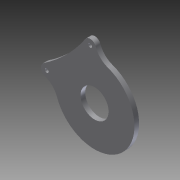
# Autodesk Inventor part: motor plate
Saved by Autodesk Inventor 2012 (Build 160160000, 160)
## iProperties
Created: 2012-02-08
Part Number: motor plate
Material: Default
Document SubType Name: Modeling
Designer: Antonella Wilby
Density: 1 g/cm^3
Author: Antonella Wilby
Autodesk Inventor part; units mm, degrees
ref_plane "YZ Plane" through (0, 0, 0) normal (1, 0, 0) x (0, 1, 0)
ref_plane "XZ Plane" through (0, 0, 0) normal (0, 1, 0) x (-1, 0, 0)
ref_plane "XY Plane" through (0, 0, 0) normal (0, 0, 1) x (1, 0, 0)
sketch "Sketch1" plane through (0, 0, 0) normal (0, 0, 1) x (1, 0, 0)
  line L0 (-237.7169, 0) -> (128.6737, 0) projected
  line L1 (0, -128.6737) -> (0, 237.7169) projected
  line L2 (0, 0) -> (-137.5064, 137.5064) construction
  circle A0 centre (0, 0) radius 19.05
  line L3 (-64.8097, 6.007) -> (-6.007, 64.8097) construction
  line L4 (0, 0) -> (-6.007, 64.8097) construction
  line L5 (0, 0) -> (-64.8097, 6.007) construction
  arc A1 (1.4866, 67.427) -> (-12.5946, 69.2377) centre (-6.007, 64.8097) ccw
  arc A2 (-69.2377, 12.5946) -> (-67.427, -1.4866) centre (-64.8097, 6.007) ccw
  circle A3 centre (-6.007, 64.8097) radius 6.35 construction
  circle A4 centre (-64.8097, 6.007) radius 6.35 construction
  arc A5 (-38.1661, 38.1661) -> (-12.5946, 69.2377) centre (-185.3754, 185.3754) ccw
  arc A6 (1.4866, 67.427) -> (17.9617, 50.8987) centre (26.9305, 76.3138) ccw
  arc A7 (-69.2377, 12.5946) -> (-38.1661, 38.1661) centre (-185.3754, 185.3754) ccw
  arc A8 (-50.8987, -17.9617) -> (-67.427, -1.4866) centre (-76.3138, -26.9305) ccw
  arc A9 (-50.8987, -17.9617) -> (17.9617, 50.8987) centre (0, 0) ccw
  point P0 (-35.4084, 35.4084)
  dimension "d1" = 45
  dimension "d2" = 38.1
  dimension "d3" = 83.1596
  dimension "d5" = 65.0875
  dimension "d6" = 12.7
  dimension "d7" = 1.5875
  dimension "d9" = 53.975
  constraints: 14 point on circle, 10 centre point, 8 coincident, 8 end point, 5 tangent, 2 equal radius, 2 point on line, 1 midpoint, 1 perpendicular, 2 other
  measures "d1" angle of L1 L2
  measures "d2" diameter of A0
  measures "d3" distance of L4.end L5.end
  measures "d5" distance of L4.start L4.end
  measures "d6" diameter of A3
  measures "d7" radial gap between concentric circles of A2 A4
  measures "d9" distance of A5.start point (0, 0)
extrude "Base" add sketch "Sketch1" along normal mid plane 6.35 contours A2 A7 A5 A1 L1 A0 L0 | L0 A0 L1 A9 A8 A2 | L1 A1 A6 A9 L0 A0 | A0 L0 A9 L1
sketch "Sketch2" plane through (0, 0, -3.175) normal (0, 0, -1) x (-1, 0, 0)
  arc A0 (12.5946, 69.2377) -> (-1.4866, 67.427) centre (6.007, 64.8097) ccw projected
  arc A1 (67.427, -1.4866) -> (69.2377, 12.5946) centre (64.8097, 6.007) ccw projected
  constraints: 2 coincident
hole "Hole1" at (-6.007, 64.8097, -3.175) at (-64.8097, 6.007, -3.175) direction (0, 0, 1) diameter 5.1054 end through all counterbore diameter 9.779 counterbore depth 1.5875 clearance for "Flat Head Machine Screw (82)" size "#10" standard "Ansi Unified Screw Threads"
body "Solid1"
